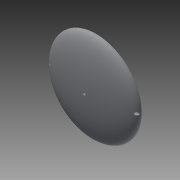
# Autodesk Inventor part: cup
Saved by Autodesk Inventor 2015 (Build 190159000, 159)
## iProperties
Created: 2019-09-28
Part Number: cup
Material: Generic
Document SubType Name: Modeling
Designer: gabri
Density: 1 g/cm^3
Appearance: Default
Author: gabri
Autodesk Inventor part; units mm, degrees
ref_plane "YZ Plane" through (0, 0, 0) normal (1, 0, 0) x (0, 1, 0)
ref_plane "XZ Plane" through (0, 0, 0) normal (0, 1, 0) x (-1, 0, 0)
ref_plane "XY Plane" through (0, 0, 0) normal (0, 0, 1) x (1, 0, 0)
sketch "Sketch4" plane through (0, 0, 0) normal (0, 0, 1) x (1, 0, 0)
  ellipse E0 centre (0, -1.5) end of major axis (-30, -1.5) minor radius 8 (-30, -1.5) -> (0, -9.5) ccw
  line L0 (0, -1.5) -> (0, -8)
  line L1 (0, -8) -> (0, -9.5)
  line L2 (-30, -1.5) -> (-28.5, -1.5)
  line L3 (28.5, -1.5) -> (30, -1.5)
  ellipse E1 centre (0, -1.5) end of major axis (-28.5, -1.5) minor radius 6.5 (-28.5, -1.5) -> (0, -8) ccw
  point P0 (0, 0)
  point P1 (0, 0)
  dimension "d15" = 60
  dimension "d19" = 6.5
  constraints: 8 end point, 3 coincident, 2 vertical, 8 other
  measures "d15" distance of L3.end L2.start
  measures "d19" distance of L0.end L0.start
revolve "Revolution2" add sketch "Sketch4" angle 360 about axis through (0, -1.5, 0) along (0, -1, 0)
sketch "Sketch5" plane through (0, -1.5, 0) normal (0, 1, 0) x (1, 0, 0)
  point P0 (0, 0)
  point P1 (0, 0)
  constraints: 1 coincident
hole "Hole2" at (0, -1.5, 0) direction (0, -1, 0) diameter 2 end through all
sketch "Sketch6" plane through (0, -1.5, 0) normal (0, 1, 0) x (1, 0, 0)
  circle A0 centre (0, 0) radius 30 projected
  circle A1 centre (0, 0) radius 28.5 projected
  line L0 (-25.0438, 10.3999) -> (-20.7015, 8.7793)
  line L1 (-24.2068, 12.2222) -> (-20.0022, 10.653)
  circle A2 centre (0, 0) radius 30 projected
  line L2 (-30, 1.5) -> (-29.8, 1.5)
  line L3 (-29.8, 1.5) -> (-29.8, -1.5)
  line L4 (-29.8, -1.5) -> (-30, -1.5)
  line L5 (-30, -1.5) -> (-30, 1.5)
  point P0 (0, 0)
  point P1 (-30, 0)
  point P2 (-28.5, 0)
  dimension "d29" = 3
  dimension "d30" = 0.2
  constraints: 12 end point, 3 horizontal alignment, 2 parallel, 1 horizontal, 1 midpoint, 1 perpendicular, 6 other
  measures "d29" distance between parallel lines of L4 L2
  measures "d30" distance between parallel lines of L5 L3
extrude "Extrusion1" cut sketch "Sketch6" against normal through all contours L2 L3 L4 A0 | A0 L5 L2 | L4 L5 A0 picked at (-29.8653, 0.1667)
sketch "Sketch7" plane through (-29.8, -1.5, -1.5) normal (-1, 0, 0) x (0, 0, 1)
  line L0 (1.5, 0) -> (1.5, -6.496) projected
  point P0 (1.5, 1.5)
  point P1 (1.5, -2)
  dimension "d33" = 2
  constraints: 1 point on line
  measures "d33" distance of L0.start point (1.5, -2)
hole "Hole3" at (-29.8, -3.5, 0) direction (1, 0, 0) diameter 2 end through all
body "Solid2"
